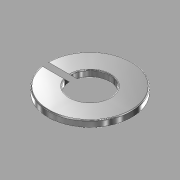
# Autodesk Inventor part: Lock Washer -2
Saved by Autodesk Inventor 2011 SP2 (Build 150309200, 309)
## iProperties
Created: 2015-02-19
Part Number: Lock Washer -2
Document SubType Name: Modeling
Designer: Greg Pavlik
Density: 1 g/cm^3
Author: Greg Pavlik
Autodesk Inventor part; units mm, degrees
ref_plane "YZ Plane" through (0, 0, 0) normal (1, 0, 0) x (0, 1, 0)
ref_plane "XZ Plane" through (0, 0, 0) normal (0, 1, 0) x (-1, 0, 0)
ref_plane "XY Plane" through (0, 0, 0) normal (0, 0, 1) x (1, 0, 0)
sketch "Sketch1" plane through (0, 0, 0) normal (0, 0, 1) x (1, 0, 0)
  circle A0 centre (0, 0) radius 4.5
  circle A1 centre (0, 0) radius 2.125
  dimension "d0" = 9
  dimension "d1" = 4.25
  constraints: 2 centre point, 1 coincident, 1 concentric
  measures "d0" diameter of A0
  measures "d1" diameter of A1
extrude "Extrusion1" add sketch "Sketch1" along normal mid plane 0.75
sketch "Sketch2" plane through (0, 0, 0) normal (1, 0, 0) x (0, 1, 0)
  line L0 (-2.125, 0.375) -> (2.125, 0.375) construction
  line L1 (2.125, -0.375) -> (-2.125, -0.375) construction
  line L2 (0, 0) -> (0, 0.375) construction
  line L3 (0, 0) -> (-0.375, 0.375) construction
  line L4 (-0.7286, 0.375) -> (0.0214, -0.375)
  line L5 (-0.0214, 0.375) -> (0.7286, -0.375)
  line L6 (0.0214, -0.375) -> (0.7286, -0.375)
  line L7 (-0.0214, 0.375) -> (-0.7286, 0.375)
  dimension "d5" = 0.5
  dimension "d9" = 45
  constraints: 12 end point, 7 point on line, 1 collinear, 1 midpoint, 1 perpendicular, 1 other
  measures "d5" distance between parallel lines of L5 L4
  measures "d9" angle of L2 L3
extrude "Extrusion2" cut sketch "Sketch2" against normal through all
fillet "Fillet1" radius 0.1 8 edges at (-0.0107, 4.5, 0.375) (0.3655, -4.4851, 0.375) (0.3655, 4.4851, -0.375) (-0.0107, -4.5, -0.375) (0.3699, -2.0926, 0.375) (-0.0107, 2.125, 0.375) (-0.0107, -2.125, -0.375) (0.3699, 2.0926, -0.375)
body "Solid1"
